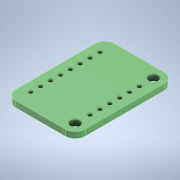
# Autodesk Inventor part: Driver_Motor
Saved by Autodesk Inventor 2022 (Build 260153000, 153)
## iProperties
Created: 2022-12-31
Part Number: Driver_Motor
Material: Generic
Document SubType Name: Modeling
Designer: karpova
Density: 1 g/cm^3
Appearance: Smooth - Dark Forest Green
Author: karpova
Autodesk Inventor part; units mm, degrees
ref_plane "YZ Plane" through (0, 0, 0) normal (1, 0, 0) x (0, 1, 0)
ref_plane "XZ Plane" through (0, 0, 0) normal (0, 1, 0) x (-1, 0, 0)
ref_plane "XY Plane" through (0, 0, 0) normal (0, 0, 1) x (1, 0, 0)
sketch "Sketch1" plane through (0, 0, 0) normal (0, 0, 1) x (1, 0, 0)
  line L0 (2.54, 0) -> (15.24, 0)
  line L1 (17.78, 2.54) -> (17.78, 22.86)
  line L2 (15.24, 25.4) -> (2.54, 25.4)
  line L3 (0, 22.86) -> (0, 2.54)
  arc A0 (17.78, 22.86) -> (15.24, 25.4) centre (15.24, 22.86) ccw
  arc A1 (15.24, 0) -> (17.78, 2.54) centre (15.24, 2.54) ccw
  arc A2 (0, 2.54) -> (2.54, 0) centre (2.54, 2.54) ccw
  arc A3 (2.54, 25.4) -> (0, 22.86) centre (2.54, 22.86) ccw
  point P0 (0, 0)
  point P1 (17.78, 25.4)
  point P2 (17.78, 0)
  point P3 (0, 25.4)
  dimension "d0" = 17.78
  dimension "d1" = 25.4
  dimension "d2" = 2.54
  constraints: 8 end point, 8 point on circle, 8 point on line, 8 tangent, 4 centre point, 3 equal radius, 2 parallel, 1 horizontal, 1 perpendicular
  measures "d0" distance of point (17.78, 25.4) point (0, 25.4)
  measures "d1" distance of point (17.78, 0) point (17.78, 25.4)
  measures "d2" radius of A0
extrude "Extrusion1" add sketch "Sketch1" along normal blind 1.5367
sketch "Sketch2" plane through (0, 0, 1.5367) normal (0, 0, 1) x (1, 0, 0)
  arc A0 (17.78, 22.86) -> (15.24, 25.4) centre (15.24, 22.86) ccw projected
  arc A1 (15.24, 0) -> (17.78, 2.54) centre (15.24, 2.54) ccw projected
  line L0 (17.78, 2.54) -> (17.78, 22.86) projected
  line L1 (15.24, 25.4) -> (2.54, 25.4) projected
  line L2 (2.54, 0) -> (15.24, 0) projected
  point P0 (0, 0)
  point P1 (15.1511, 22.7711)
  point P2 (15.1511, 2.6289)
  dimension "d36" = 2.6289
  dimension "d37" = 2.6289
  dimension "d38" = 2.6289
  dimension "d39" = 2.6289
  measures "d36" distance from line of point (15.151, 22.771) L0
  measures "d37" distance from line of point (15.151, 22.771) L1
  measures "d38" distance from line of point (15.151, 2.629) L0
  measures "d39" distance from line of point (15.151, 2.629) L2
hole "Hole1" at (15.1511, 22.7711, 1.5367) at (15.1511, 2.6289, 1.5367) direction (0, 0, -1) diameter 2.4638 end through all both
sketch "Sketch3" plane through (0, 0, 1.5367) normal (0, 0, 1) x (1, 0, 0)
  arc A0 (17.78, 22.86) -> (15.24, 25.4) centre (15.24, 22.86) ccw construction
  line L0 (15.24, 25.4) -> (15.24, 0) construction
  arc A1 (15.24, 0) -> (17.78, 2.54) centre (15.24, 2.54) ccw construction
  line L1 (2.54, 0) -> (15.24, 0) construction
  line L2 (15.24, 25.4) -> (2.54, 25.4) construction
  line L3 (2.54, 0) -> (2.54, 25.4) construction
  line L4 (0, 22.86) -> (0, 2.54) construction
  line L5 (0, 12.7) -> (17.78, 12.7) construction
  line L6 (17.78, 2.54) -> (17.78, 22.86) construction
  line L7 (8.89, 25.4) -> (8.89, 0) construction
  point P0 (0, 0)
  point P1 (15.24, 13.97)
  point P2 (2.54, 13.97)
  point P3 (15.24, 16.51)
  point P4 (15.24, 19.05)
  point P5 (15.24, 11.43)
  point P6 (15.24, 13.97)
  point P7 (15.24, 16.51)
  point P8 (15.24, 8.89)
  point P9 (15.24, 11.43)
  point P10 (15.24, 13.97)
  point P11 (15.24, 6.35)
  point P12 (15.24, 8.89)
  point P13 (15.24, 11.43)
  point P14 (2.54, 16.51)
  point P15 (2.54, 19.05)
  point P16 (2.54, 21.59)
  point P17 (2.54, 11.43)
  point P18 (2.54, 13.97)
  point P19 (2.54, 16.51)
  point P20 (2.54, 19.05)
  point P21 (2.54, 8.89)
  point P22 (2.54, 11.43)
  point P23 (2.54, 13.97)
  point P24 (2.54, 16.51)
  point P25 (2.54, 6.35)
  point P26 (2.54, 8.89)
  point P27 (2.54, 11.43)
  point P28 (2.54, 13.97)
  point P29 (2.54, 3.81)
  point P30 (2.54, 6.35)
  point P31 (2.54, 8.89)
  point P32 (2.54, 11.43)
  dimension "d12" = 1.27
  dimension "d15" = 2.54
  dimension "d18" = 2.54
  dimension "d23" = 2.54
  dimension "d26" = 2.54
  constraints: 8 end point, 5 vertical, 4 midpoint, 1 point on circle, 1 point on line, 1 symmetric about line, 30 other
  measures "d12" distance from line of L5 point (15.24, 13.97)
  measures "d15" distance of point (15.24, 13.97) point (15.24, 16.51)
  measures "d18" distance of point (15.24, 13.97) point (15.24, 11.43)
  measures "d23" distance of point (2.54, 13.97) point (2.54, 16.51)
  measures "d26" distance of point (2.54, 13.97) point (2.54, 11.43)
hole "Hole2" at (15.24, 13.97, 1.5367) at (2.54, 13.97, 1.5367) at (15.24, 16.51, 1.5367) at (15.24, 19.05, 1.5367) at (15.24, 11.43, 1.5367) at (15.24, 8.89, 1.5367) at (15.24, 6.35, 1.5367) at (2.54, 16.51, 1.5367) at (2.54, 19.05, 1.5367) at (2.54, 21.59, 1.5367) at (2.54, 11.43, 1.5367) at (2.54, 8.89, 1.5367) at (2.54, 6.35, 1.5367) at (2.54, 3.81, 1.5367) direction (0, 0, -1) diameter 1.016 end through all both
equation "\"d3\" = pcbThickness"
equation "\"d5\" = mountingHoleDiameter"
equation "\"d12\" = 0.5 * pinHoleSeparationDistance"
equation "\"d15\" = pinHoleSeparationDistance"
equation "\"d18\" = pinHoleSeparationDistance"
equation "\"d23\" = pinHoleSeparationDistance"
equation "\"d26\" = pinHoleSeparationDistance"
equation "\"d29\" = pinHoleDiameter"
equation "\"pcbThickness\" = 1.5367"
equation "\"mountingHoleDiameter\" = 2.4638"
equation "\"pinHoleDiameter\" = 1.016"
equation "\"pinHoleSeparationDistance\" = 2.54"
body "Solid1"
